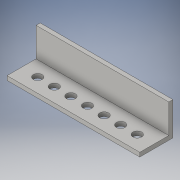
# Autodesk Inventor part: 4 L aluminum piece for transmission bracket
Saved by Autodesk Inventor 2016 SP2 (Build 200236200, 236)
## iProperties
Created: 2018-02-04
Part Number: 4 L aluminum piece for transmission bracket
Material: Generic
Document SubType Name: Modeling
Designer: CAD
Density: 1 g/cm^3
Appearance: Default
Author: CAD
Autodesk Inventor part; units mm, degrees
ref_plane "YZ Plane" through (0, 0, 0) normal (1, 0, 0) x (0, 1, 0)
ref_plane "XZ Plane" through (0, 0, 0) normal (0, 1, 0) x (-1, 0, 0)
ref_plane "XY Plane" through (0, 0, 0) normal (0, 0, 1) x (1, 0, 0)
sketch "Sketch1" plane through (0, 0, 0) normal (0, 0, 1) x (1, 0, 0)
  line L0 (0, 0) -> (101.6, 0)
  line L1 (101.6, 0) -> (101.6, 25.4)
  line L2 (101.6, 25.4) -> (0, 25.4)
  line L3 (0, 25.4) -> (0, 0)
  dimension "d0" = 101.6
  dimension "d1" = 25.4
  constraints: 8 end point, 2 parallel, 1 horizontal, 1 perpendicular
  measures "d0" distance of L2.end L1.end
  measures "d1" distance of L0.end L1.end
extrude "Extrusion1" add sketch "Sketch1" along normal blind 3.175
sketch "Sketch2" plane through (0, 0, 3.175) normal (0, 0, 1) x (1, 0, 0)
  line L0 (0, 0) -> (101.6, 0) projected
  line L1 (0, 0) -> (101.6, 0)
  line L2 (101.6, 0) -> (101.6, 3.175)
  line L3 (101.6, 0) -> (101.6, 25.4) projected
  line L4 (101.6, 3.175) -> (0, 3.175)
  line L5 (0, 3.175) -> (0, 0)
  dimension "d4" = 3.175
  constraints: 8 end point, 2 perpendicular, 1 collinear, 1 point on line
  measures "d4" distance of L0.end L2.end
extrude "Extrusion2" add sketch "Sketch2" along normal blind 22.225
sketch "Sketch3" plane through (0, 0, 0) normal (0, -1, 0) x (1, 0, 0)
  line L0 (0, 0) -> (0, 25.4) projected
  line L1 (101.6, 0) -> (101.6, 25.4) projected
  line L2 (0, 0) -> (101.6, 0) projected
  point P0 (12.7, 14.605)
  point P1 (25.4, 14.605)
  point P2 (38.1, 14.605)
  point P3 (50.8, 14.605)
  point P4 (63.5, 14.605)
  point P5 (76.2, 14.605)
  point P6 (88.9, 14.605)
  dimension "d7" = 12.7
  dimension "d9" = 12.7
  dimension "d10" = 12.7
  dimension "d11" = 12.7
  dimension "d12" = 12.7
  dimension "d13" = 12.7
  dimension "d14" = 12.7
  dimension "d15" = 14.605
  dimension "d16" = 14.605
  dimension "d17" = 14.605
  dimension "d18" = 14.605
  dimension "d19" = 14.605
  dimension "d20" = 14.605
  dimension "d21" = 14.605
  measures "d7" distance from line of L0 point (12.7, 14.605)
  measures "d9" distance of point (38.1, 14.605) point (25.4, 14.605)
  measures "d10" distance of point (50.8, 14.605) point (38.1, 14.605)
  measures "d11" distance of point (63.5, 14.605) point (50.8, 14.605)
  measures "d12" distance of point (76.2, 14.605) point (63.5, 14.605)
  measures "d13" distance of point (88.9, 14.605) point (76.2, 14.605)
  measures "d14" distance from line of L1 point (88.9, 14.605)
  measures "d15" distance from line of L2 point (12.7, 14.605)
  measures "d16" distance from line of L2 point (25.4, 14.605)
  measures "d17" distance from line of L2 point (38.1, 14.605)
  measures "d18" distance from line of L2 point (50.8, 14.605)
  measures "d19" distance from line of L2 point (63.5, 14.605)
  measures "d20" distance from line of L2 point (76.2, 14.605)
  measures "d21" distance from line of L2 point (88.9, 14.605)
hole "Hole1" at (12.7, 0, 14.605) at (25.4, 0, 14.605) at (38.1, 0, 14.605) at (50.8, 0, 14.605) at (63.5, 0, 14.605) at (76.2, 0, 14.605) at (88.9, 0, 14.605) direction (0, 1, 0) diameter 6.731 depth 25.4 tip angle 118
body "Solid1"
